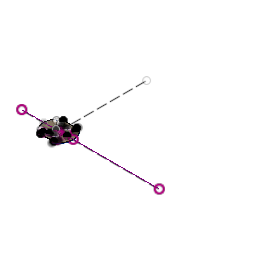
E yantra v1 (Autodesk Fusion 360 design; units mm, degrees)
Autodesk Fusion 360 part; units mm, degrees
note: some values were not read from the file. Set by a fixed rule: which sketch regions a step uses.
sketch "Sketch1" plane through (0, 0, 0) normal (0, 1, 0) x (1, 0, 0)
  line L0 (-45, 60) -> (45, 60)
  line L1 (45, 60) -> (45, 90)
  line L2 (-45, 60) -> (-45, 90)
  line L3 (0, 0) -> (685.6072, 0) construction
  line L4 (45, -60) -> (45, -90)
  line L5 (-45, -60) -> (-45, -90)
  line L6 (-45, -60) -> (45, -60)
  line L7 (0, 0) -> (0, 600) construction
  line L8 (0, 0) -> (-250, 0) construction
  arc A0 (-45, 90) -> (-45, -90) centre (1.1364, 0) ccw
  arc A1 (45, -90) -> (45, 90) centre (-1.1364, 0) ccw
  line L9 (25, 17.5) -> (37, 17.5)
  line L10 (37, 17.5) -> (37, -17.5)
  line L11 (37, -17.5) -> (25, -17.5)
  line L12 (25, -17.5) -> (25, 17.5)
  dimension "d1" = 45
  dimension "d2" = 45
  dimension "d3" = 120
  dimension "d4" = 30
  dimension "d5" = 100
  dimension "d8" = 70
  dimension "d9" = 12
  dimension "d10" = 35
  measures "d1" distance of L2 L7
  measures "d2" distance of L1 L7
  measures "d3" distance of L0 L6
  measures "d8" distance of L5 L12
extrude "Extrude1" add sketch "Sketch1" along normal blind 4 contours L0 L1 L2 L4 L5 L6 A0 A1 | L9 L10 L11 L12 makes body 1
extrude "Extrude2" cut sketch "Sketch1" along normal up to surface (4 mm away) contours L9 L10 L11 L12 bodies 1
copy_body "CopyPasteBodies1" bodies 1 makes body 2
move_body "Move1" bodies 2 to x (1, 0, 0) y (0, 1, 0) z (0, 0, 1) at (0, 44, 0)
sketch "Sketch2" plane through (0, 48, 0) normal (0, 1, 0) x (-1, 0, 0)
  line L0 (-37, -17.5) -> (-37, 17.5)
  line L1 (-37, 17.5) -> (-25, 17.5)
  line L2 (-25, 17.5) -> (-25, -17.5)
  line L3 (-25, -17.5) -> (-37, -17.5)
  line L4 (45, 60) -> (-45, 60)
  line L5 (-45, 60) -> (-45, 90)
  arc A0 (-45, 90) -> (-45, -90) centre (1.1364, 0) ccw
  line L6 (-45, -90) -> (-45, -60)
  line L7 (-45, -60) -> (45, -60)
  line L8 (45, -60) -> (45, -90)
  arc A1 (45, -90) -> (45, 90) centre (-1.1364, 0) ccw
  line L9 (45, 90) -> (45, 60)
  line L10 (45, -90) -> (-45, -90)
  line L11 (45, 90) -> (-45, 90)
  line L12 (100, 0) -> (70, 0) construction
  line L13 (70, 0) -> (70, -20)
  line L14 (70, 0) -> (70, 20)
  line L15 (70, 20) -> (98.0028, 20)
  line L16 (70, -20) -> (98.0028, -20)
  line L17 (-55, 0) -> (-55, -12) construction
  circle A2 centre (-55, -12) radius 17.5
  line L18 (-55, -12) -> (-55, -29.5) construction
  line L19 (-55, -29.5) -> (-95.602, -29.5)
  line L20 (-55, 5.5) -> (-99.8503, 5.5)
  line L21 (-99.8503, 5.5) -> (-99.8503, 90)
  line L22 (-99.8503, 90) -> (-45, 90)
  dimension "d17" = 30
  dimension "d18" = 20
  dimension "d19" = 20
  dimension "d22" = 12
  dimension "d23" = 45
  dimension "d24" = 35
  measures "d22" distance of origin
  measures "d24" diameter of A2
extrude "Extrude7" add sketch "Sketch2" against normal blind 4 contours A0 L21 L22 bodies 2
extrude "Extrude6" cut sketch "Sketch2" against normal up to surface (4 mm away) contours A0 A2 L19 L20 | A2 bodies 2
extrude "Extrude3" add sketch "Sketch2" against normal blind 4 contours L4 L5 L9 L11 | L6 L7 L8 L10 bodies 2
extrude "Extrude4" add 1 faces at (37, 46.6667, -5.8333) along direction (-1, 0, 0) up to surface (12 mm away) on bodies 2 bodies 2
extrude "Extrude5" cut sketch "Sketch2" against normal up to surface (4 mm away) contours A1 L13 L14 L15 L16 bodies 2
fillet "Fillet1" radius 20 1 edges at (99.8503, 46, 90) on bodies 2
sketch "Sketch3" plane through (0, 4, 0) normal (0, 1, 0) x (-1, 0, 0)
  line L0 (-37, -17.5) -> (-37, 17.5)
  line L1 (-37, 17.5) -> (-25, 17.5)
  line L2 (-25, 17.5) -> (-25, -17.5)
  line L3 (-25, -17.5) -> (-37, -17.5)
  line L4 (45, 60) -> (-45, 60)
  line L5 (-45, 60) -> (-45, 90)
  arc A0 (-45, 90) -> (-45, -90) centre (1.1364, 0) ccw
  line L6 (-45, -90) -> (-45, -60)
  line L7 (-45, -60) -> (45, -60)
  line L8 (45, -60) -> (45, -90)
  arc A1 (45, -90) -> (45, 90) centre (-1.1364, 0) ccw
  line L9 (45, 90) -> (45, 60)
  line L10 (45, 60) -> (4, 60) construction
  line L11 (4, 60) -> (4, 41) construction
  line L12 (4, 41) -> (18.25, 41) construction
  circle A2 centre (18.25, 41) radius 1.5
  circle A3 centre (-10.25, 41) radius 1.5
  line L13 (0, 0) -> (250, 0)
  line L14 (0, 0) -> (17.4328, 0) construction
  circle A4 centre (18.25, -41) radius 1.5
  circle A5 centre (-10.25, -41) radius 1.5
  line L15 (0, 0) -> (-685.6072, 0)
  line L16 (45, 60) -> (-45, 60)
  line L17 (45, -78) -> (-45, -78)
  line L18 (45, 78) -> (-45, 78)
  line L19 (-58.3939, 0) -> (-58.3939, -57) construction
  circle A6 centre (-58.3939, -57) radius 1.5
  circle A7 centre (-58.3939, 57) radius 1.5
  line L20 (-37, -17.5) -> (-37, 17.5)
  circle A8 centre (-22, -41) radius 1.5
  circle A9 centre (-22, 41) radius 1.5
  circle A10 centre (66.3533, 53.4338) radius 1.5
  circle A11 centre (66.3533, -53.4338) radius 1.5
  circle A12 centre (35.6432, -48.7943) radius 1.5
  circle A13 centre (35.6432, 48.7943) radius 1.5
  dimension "d30" = 41
  dimension "d32" = 14.25
  dimension "d33" = 3
  dimension "d38" = 19
  dimension "d40" = 78
  dimension "d43" = 57
  dimension "d44" = 41.6061
  dimension "d45" = 3
  dimension "d47" = 63
  dimension "d48" = 3
  dimension "d49" = 3
  dimension "d50" = 3
  measures "d30" distance of L13.start
  measures "d33" diameter of A2
  measures "d38" distance of L10 L12
  measures "d40" distance of L14 L17
  measures "d45" diameter of A6
  measures "d47" distance of L13.start L20
  measures "d48" diameter of A8
  measures "d49" diameter of A10
  measures "d50" diameter of A12
extrude "Extrude10" cut sketch "Sketch3" along normal blind -70 and the other way blind -190 contours A6 | A7 | A8 | A9 | A10 | A11 | A12 | A13 bodies 1 2
extrude "Extrude8" add sketch "Sketch3" against normal blind 4 contours L4 L5 L9 L16 L18 | L6 L7 L8 L17 bodies 1
move_body "Move2" bodies 2 to x (1, 0, 0) y (0, 1, 0) z (0, 0, 1) at (0, -10, 0)
hidden bodies 2
equation "d2 = d1"
equation "d8 = 83 mm - 8 mm - 5 mm"
equation "d23 = 10 mm + 35 mm"
equation "d32 = ( 28.5 / 2 ) * 1 mm"
